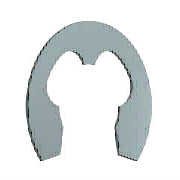
# Autodesk Inventor part: ANSI B27.7 - 5, E
Saved by Autodesk Inventor 2020.2 (Build 242310000, 310)
## iProperties
Created: 2019-01-20
Part Number: ANSI B27.7 - 5, E
Material: Steel, Mild
Description: General Purpose Tappered and Reduced Cross Section Retaining Rings - E-Ring External Series 3CM1 Retaining Rings
Document SubType Name: Modeling
Standard: ANSI B27.7
Designer: james
Standard Revision: 1999
Standards Organization: ANSI
Language: en-US
Size Designation: 5
Categories: <MemberInstance><Categories><Category DisplayName="Shaft Parts" InternalName="7f7aeb1f-a693-4053-b835-cee3144e0d98" Mnemonic="SHFT"><Category DisplayName="Circlips" InternalName="413b042a-1f46-4051-a560-0e0e417af91f" Mnemonic="CLIP"><CategoryParameter DisplayName="Thickness" InternalName="230c7f7c-2544-4c6d-b8d5-773e831b23fa" Mnemonic="thick"/><CategoryParameter DisplayName="Groove Diameter" InternalName="4054b45c-161d-4ad6-befb-f30b3855ce84" Mnemonic="grvdia"/><CategoryParameter DisplayName="Groove Width" InternalName="4dde6996-4bf1-443b-8317-d4f4fc6b9be0" Mnemonic="NB"/><CategoryParameter DisplayName="Shaft Diameter" InternalName="a433c9ab-b9eb-4798-a453-f2210a67728e" Mnemonic="shaftdia"/><Category DisplayName="External" InternalName="a9a2b132-a8be-48ab-9c3d-0c324a909558" Mnemonic="OUCLIP"><CategoryParameter DisplayName="Shaft Diameter Min." InternalName="62b77b9b-1e86-4b9a-9911-d7c0fa48fc9a" Mnemonic="shaftdiamin"/><CategoryParameter DisplayName="Outer Diameter" InternalName="a3599e7b-be7c-41b5-9a50-6dab253b0906" Mnemonic="outdia"/></Category></Category></Category><Category DisplayName="DataType" InternalName="23b78d0f-2648-40c6-8793-ca6db495c9e8" Mnemonic="DATATYPE"><CategoryParameter DisplayName="DisplayName" InternalName="05415f3d-3907-474b-a020-eb9d644f4cf3" Mnemonic="DISPLAYNAME"/><CategoryParameter DisplayName="Standard" InternalName="0c0a119c-1e12-4c84-803f-101930972f5e" Mnemonic="STANDARD"/><CategoryParameter DisplayName="Description" InternalName="13903e3d-64b1-4950-80da-f627842ea37f" Mnemonic="DESCRIPTION"/><CategoryParameter DisplayName="Designation" InternalName="2675968c-4ce5-49e0-a4f5-552d29089031" Mnemonic="DESIGNATION"/><CategoryParameter DisplayName="Default Row" InternalName="2af9ec52-faaa-4026-b378-f9fa4afca842" Mnemonic="DEFAULTROW"/><CategoryParameter DisplayName="Folder Name" InternalName="3f06958e-8713-4116-9be7-ed6184ecc97b" Mnemonic="FOLDERNAME"/><CategoryParameter DisplayName="Revision Guid" InternalName="45a75005-10b1-4dfc-8d6d-dfe629f0b93c" Mnemonic="REVISIONGUID"/><CategoryParameter DisplayName="FileName" InternalName="8b46a4cc-9585-4fed-90c3-899f57e09a73" Mnemonic="FILENAME"/><CategoryParameter DisplayName="StdsOrg" InternalName="8f5914e1-4693-403f-8ab5-d37768198c9d" Mnemonic="STDSORG"/><CategoryParameter DisplayName="Family Version" InternalName="914462f6-6e19-4b14-ba84-155b9680b1d0" Mnemonic="FAMILYREVISION"/><CategoryParameter DisplayName="Standard Revision" InternalName="91d5a463-65c2-4fde-b823-3b7fea5e8e17" Mnemonic="STANDARDREVISION"/><CategoryParameter DisplayName="Member Revision" InternalName="a65d44b9-392f-4f4f-857b-e4b3d54996fe" Mnemonic="MEMBERREVISION"/><CategoryParameter DisplayName="ClipFormat" InternalName="bc51e27b-3422-4e78-93ef-cec197ddf230" Mnemonic="CLIPFORMAT"/><CategoryParameter DisplayName="Manufacturer" InternalName="cd6c7a72-a28a-4e50-99a9-2c7f4e13e5ad" Mnemonic="MANUFACTURER"/><CategoryParameter DisplayName="InternalName" InternalName="cf1d0246-76d9-4b4a-8305-fa0409afb5c1" Mnemonic="INTERNALNAME"/><CategoryParameter DisplayName="IsMetric" InternalName="e2385c5b-1ea4-4823-96a8-8de651266ec3" Mnemonic="ISMETRIC"/><Category DisplayName="Part" InternalName="c0e0b642-3bcb-4cc8-9e80-f96d35c4afa4" Mnemonic="PART"><CategoryParameter DisplayName="Part Number" InternalName="016b6077-bfbe-49bd-92c9-d8d59c39c941" Mnemonic="PARTNUMBER"/><CategoryParameter DisplayName="Stock Number" InternalName="4dba7c1c-e26c-444e-836c-b08b433409a8" Mnemonic="STOCKNUMBER"/><CategoryParameter DisplayName="Material Key" InternalName="5c9a8adb-dd2b-4535-b97f-0a94a95fe41f" Mnemonic="MATERIALKEY"/><CategoryParameter DisplayName="Material" InternalName="818a152a-d3c3-49ca-80ee-df7d91421b8e" Mnemonic="MATERIAL"/></Category></Category><Category DisplayName="LegacyMap" InternalName="cd87c42b-3e48-431e-b5c0-1cbeb14dfe77" Mnemonic="LEGACYMAP"><CategoryParameter DisplayName="unique DA member ID" InternalName="0918ad47-427f-4fed-ae26-24c81c58f590" Mnemonic="DACOOKIE"/><CategoryParameter DisplayName="Merge11 ID" InternalName="0ee8fb18-e2ed-4f39-96f6-1f4b5f50aa71" Mnemonic="MERGE11"/><CategoryParameter DisplayName="unique CC member ID" InternalName="5193edd4-b2b0-4ab4-9d54-de900eee34e0" Mnemonic="CCCOOKIE"/><CategoryParameter DisplayName="Split ID" InternalName="72b5c83c-be7f-45c4-ae51-9160ea6deb26" Mnemonic="SPLIT"/><CategoryParameter DisplayName="MemberID" InternalName="8e5e0294-fc51-4c8f-b3d7-003dc5ed94f6" Mnemonic="MEMBERID"/><CategoryParameter DisplayName="CatalogName" InternalName="d99d1e27-aa94-4de2-af4c-c348882a6f4f" Mnemonic="CATALOGNAME"/><CategoryParameter DisplayName="FamilyNumber" InternalName="e705e1f4-09cb-413e-91f9-551b4188271e" Mnemonic="FAMILYNUMBER"/></Category></Categories><FamilyTemplate Id="si0132"><FamilyTemplateParameters><FamilyTemplateParameter ObjectType="kUserParameterObject" ValueType="xs:double" Id="1" ObjectReferenceKey="WDMIN"/><FamilyTemplateParameter ObjectType="kUserParameterObject" ValueType="xs:double" Id="2" ObjectReferenceKey="SNB"/><FamilyTemplateParameter ObjectType="kUserParameterObject" ValueType="xs:double" Id="3" ObjectReferenceKey="SD2"/><FamilyTemplateParameter ObjectType="kUserParameterObject" ValueType="xs:double" Id="4" ObjectReferenceKey="SD"/><FamilyTemplateParameter ObjectType="kUserParameterObject" ValueType="xs:double" Id="5" ObjectReferenceKey="ND"/><FamilyTemplateParameter ObjectType="kUserParameterObject" ValueType="xs:double" Id="6" ObjectReferenceKey="WDMAX"/><FamilyTemplateParameter ObjectType="kUserParameterObject" ValueType="xs:double" Id="7" ObjectReferenceKey="BUBRMI"/><FamilyTemplateParameter ObjectType="kUserParameterObject" ValueType="xs:double" Id="8" ObjectReferenceKey="WD"/><FamilyTemplateParameter ObjectType="kPropertyObject" ValueType="xs:string" Id="100" ObjectReferenceKey="{32853F0F-3444-11d1-9E93-0060B03C1CA6}" SubObjectId="52"/><FamilyTemplateParameter ObjectType="kPropertyObject" ValueType="xs:string" Id="105" ObjectReferenceKey="{32853F0F-3444-11d1-9E93-0060B03C1CA6}" SubObjectId="5"/><FamilyTemplateParameter ObjectType="kPartComponentDefinitionObject" ValueType="xs:string" Id="110" SubObjectId="Material"/></FamilyTemplateParameters></FamilyTemplate><CategoryParameterMap><ParamToTemplateMap><ParamToTemplate CategoryParameter="//CategoryParameter[@InternalName='05415f3d-3907-474b-a020-eb9d644f4cf3']" ConstantValue="E-Ring"/><ParamToTemplate CategoryParameter="//CategoryParameter[@InternalName='cf1d0246-76d9-4b4a-8305-fa0409afb5c1']" ConstantValue="b2abae67-a060-4369-a73f-bfa9c109ed2b"/><ParamToTemplate CategoryParameter="//CategoryParameter[@InternalName='3f06958e-8713-4116-9be7-ed6184ecc97b']" ConstantValue="ANSI B27.7(1)"/><ParamToTemplate CategoryParameter="//CategoryParameter[@InternalName='914462f6-6e19-4b14-ba84-155b9680b1d0']" ConstantValue="10"/><ParamToTemplate CategoryParameter="//CategoryParameter[@InternalName='bc51e27b-3422-4e78-93ef-cec197ddf230']" ConstantValue="CF_INVENTOR.STDPARTS"/><ParamToTemplate CategoryParameter="//CategoryParameter[@InternalName='e2385c5b-1ea4-4823-96a8-8de651266ec3']" ConstantValue="true"/><ParamToTemplate CategoryParameter="//CategoryParameter[@InternalName='13903e3d-64b1-4950-80da-f627842ea37f']" ConstantValue="General Purpose Tappered and Reduced Cross Section Retaining Rings - E-Ring External Series 3CM1 Retaining Rings"/><ParamToTemplate CategoryParameter="//CategoryParameter[@InternalName='8f5914e1-4693-403f-8ab5-d37768198c9d']" ConstantValue="ANSI"/><ParamToTemplate CategoryParameter="//CategoryParameter[@InternalName='0c0a119c-1e12-4c84-803f-101930972f5e']" ConstantValue="ANSI B27.7"/><ParamToTemplate CategoryParameter="//CategoryParameter[@InternalName='cd6c7a72-a28a-4e50-99a9-2c7f4e13e5ad']" TemplateParameter="104"/><ParamToTemplate CategoryParameter="//CategoryParameter[@InternalName='91d5a463-65c2-4fde-b823-3b7fea5e8e17']" ConstantValue="1999"/><ParamToTemplate CategoryParameter="//CategoryParameter[@InternalName='45a75005-10b1-4dfc-8d6d-dfe629f0b93c']" ConstantValue="03a39f5a-cc79-4db4-a1e3-575c0a13520e"/><ParamToTemplate CategoryParameter="//CategoryParameter[@InternalName='2af9ec52-faaa-4026-b378-f9fa4afca842']" ConstantValue="10"/><ParamToTemplate CategoryParameter="//CategoryParameter[@InternalName='d99d1e27-aa94-4de2-af4c-c348882a6f4f']" ConstantValue="ANSI"/><ParamToTemplate CategoryParameter="//CategoryParameter[@InternalName='e705e1f4-09cb-413e-91f9-551b4188271e']" ConstantValue="1254"/><ParamToTemplate CategoryParameter="//CategoryParameter[@InternalName='8b46a4cc-9585-4fed-90c3-899f57e09a73']" ConstantValue="ANSI B27.7 - 53.9(1)"/><ParamToTemplate CategoryParameter="//CategoryParameter[@InternalName='a65d44b9-392f-4f4f-857b-e4b3d54996fe']" ConstantValue="43911896-F686-47C9-83D5-A922659F7077"/><ParamToTemplate CategoryParameter="//CategoryParameter[@InternalName='8e5e0294-fc51-4c8f-b3d7-003dc5ed94f6']" ConstantValue="50"/><ParamToTemplate CategoryParameter="//CategoryParameter[@InternalName='2675968c-4ce5-49e0-a4f5-552d29089031']" TemplateParameter="100"/><ParamToTemplate CategoryParameter="//CategoryParameter[@InternalName='818a152a-d3c3-49ca-80ee-df7d91421b8e']" TemplateParameter="110"/><ParamToTemplate CategoryParameter="//CategoryParameter[@InternalName='4054b45c-161d-4ad6-befb-f30b3855ce84']" TemplateParameter="5"/><ParamToTemplate CategoryParameter="//CategoryParameter[@InternalName='016b6077-bfbe-49bd-92c9-d8d59c39c941']" TemplateParameter="105"/><ParamToTemplate CategoryParameter="//CategoryParameter[@InternalName='230c7f7c-2544-4c6d-b8d5-773e831b23fa']" TemplateParameter="4"/><ParamToTemplate CategoryParameter="//CategoryParameter[@InternalName='4dde6996-4bf1-443b-8317-d4f4fc6b9be0']" TemplateParameter="2"/><ParamToTemplate CategoryParameter="//CategoryParameter[@InternalName='a433c9ab-b9eb-4798-a453-f2210a67728e']" TemplateParameter="8"/><ParamToTemplate CategoryParameter="//CategoryParameter[@InternalName='62b77b9b-1e86-4b9a-9911-d7c0fa48fc9a']" TemplateParameter="1"/></ParamToTemplateMap></CategoryParameterMap></MemberInstance>
Density: 7.85 g/cm^3
Appearance: Semi-Polished
Mass: 0.123867 g
Surface Area: 0.760929 cm^2
Volume: 0.0157793 cm^3
IsCustomPart: 0
Author: james
Autodesk Inventor part; units mm, degrees
ref_plane "YZ Plane" through (0, 0, 0) normal (1, 0, 0) x (0, 1, 0)
ref_plane "XZ Plane" through (0, 0, 0) normal (0, 1, 0) x (-1, 0, 0)
sketch "Sketch1" plane through (0, 0, 0) normal (0, 0, 1) x (1, 0, 0)
  circle A0 centre (0, -2.4764) radius 2.5 construction
  line L0 (-0.39, 0.0236) -> (0, 0.0236) construction
  line L1 (-3.206, 0) -> (3.4858, 0) projected
  line L2 (-1.7872, -3.2564) -> (1.7872, -3.2564) construction
  arc A1 (-1.847, -1.8509) -> (-1.7872, -3.2564) centre (0, -2.4764) ccw
  line L3 (0, 1.949) -> (0, -3.4788) projected
  arc A2 (-0.39, -0.1364) -> (0.39, -0.1364) centre (0, -0.1364) ccw
  arc A3 (3.3844, -5.047) -> (-3.3844, -5.047) centre (0, -2.4764) ccw
  line L4 (-2.34, -1.6964) -> (-1.9578, -1.6964)
  line L5 (-0.39, -0.1364) -> (-0.39, 0.2425)
  arc A4 (-0.78, 0.5446) -> (-2.7529, -1.0081) centre (0, -2.4764) ccw
  arc A5 (-0.39, 0.2425) -> (-0.78, 0.5446) centre (-0.702, 0.2425) ccw
  arc A6 (-2.7529, -1.0081) -> (-2.34, -1.6964) centre (-2.34, -1.2284) ccw
  arc A7 (-1.847, -1.8509) -> (-1.9578, -1.6964) centre (-1.9578, -1.8134) ccw
  line L6 (0, 1.7736) -> (2.5298, 1.7736) construction
  line L7 (-1.7872, -3.2564) -> (-2.3673, -4.889)
  arc A8 (-3.3844, -5.047) -> (-2.3673, -4.889) centre (-2.9185, -4.6932) ccw
  line L8 (0, -0.5264) -> (-1.2778, -0.5264) construction
  line L9 (1.7872, -3.2564) -> (2.3673, -4.889)
  arc A9 (2.3673, -4.889) -> (3.3844, -5.047) centre (2.9185, -4.6932) ccw
  arc A10 (1.7872, -3.2564) -> (1.847, -1.8509) centre (0, -2.4764) ccw
  line L10 (2.34, -1.6964) -> (1.9578, -1.6964)
  line L11 (0.39, -0.1364) -> (0.39, 0.2425)
  arc A11 (2.7529, -1.0081) -> (0.78, 0.5446) centre (0, -2.4764) ccw
  arc A12 (0.78, 0.5446) -> (0.39, 0.2425) centre (0.702, 0.2425) ccw
  arc A13 (2.34, -1.6964) -> (2.7529, -1.0081) centre (2.34, -1.2284) ccw
  arc A14 (1.9578, -1.6964) -> (1.847, -1.8509) centre (1.9578, -1.8134) ccw
  point P0 (0.39, 0.0236)
  dimension "d0" = 5
  dimension "d3" = 0.78
  dimension "d4" = 0.39
  dimension "d5" = 8.5
  dimension "d8" = 3.12
  dimension "d9" = 0.78
  dimension "d10" = 0.312
  dimension "d11" = 0.468
  dimension "d12" = 0.117
  dimension "d13" = 0.585
  dimension "d14" = 1.95
  dimension "d15" = 1.95
  constraints: 30 point on circle, 20 end point, 15 centre point, 13 symmetric about line, 12 tangent, 8 point on line, 4 parallel, 2 coincident, 2 horizontal, 1 concentric, 1 perpendicular, 1 vertical alignment, 9 other
  measures "d0" diameter of A0
  measures "d3" distance from line of A1.centre L2
  measures "d4" radius of A2
  measures "d5" diameter of A3
  measures "d8" radius of A4
  measures "d9" distance from line of A1.centre L4
  measures "d10" radius of A5
  measures "d11" radius of A6
  measures "d12" radius of A7
  measures "d13" radius of A8
  measures "d14" distance from line of A1.centre L8
  measures "d15" radius of A1
extrude "Body" add sketch "Sketch1" along normal blind 0.6 contours A4 A6 L4 A7 A1 L7 A8 A3 L3 L1 L5 A5 | L1 L3 A2 L5 | L3 A3 L1 A11 A12 L11 | L1 L11 A2 L3 | L1 A3 A9 L9 A10 A14 L10 A13 A11
ref_plane "Work Plane1" through (0, -2.4764, 0) normal (-1, 0, 0) x (0, 0, 1)
equation "\"d0\" = WD"
equation "\"d3\" = 0.2 * ND"
equation "\"d4\" = 0.1 * ND"
equation "\"d5\" = SD2"
equation "\"d8\" = 0.8 * ND"
equation "\"d9\" = 0.2 * ND"
equation "\"d10\" = 0.08 * ND"
equation "\"d11\" = 0.12 * ND"
equation "\"d12\" = 0.03 * ND"
equation "\"d13\" = 0.15 * ND"
equation "\"d14\" = 0.5 * ND"
equation "\"d15\" = 0.5 * ND"
equation "\"d16\" = SD"
equation "\"ND\" = 3.9"
equation "\"SD\" = 0.6"
equation "\"WD\" = WDMIN"
equation "\"d1\" = 1.6 * ND"
equation "\"d2\" = ND"
equation "\"SD2\" = 8.5"
equation "\"d6\" = ND"
equation "\"d7\" = 0.15 * ND"
equation "\"WDMIN\" = 5"
equation "\"SNB\" = 0.7"
equation "\"WDMAX\" = 6"
equation "\"BUBRMI\" = 1.1"
body "Solid1"
